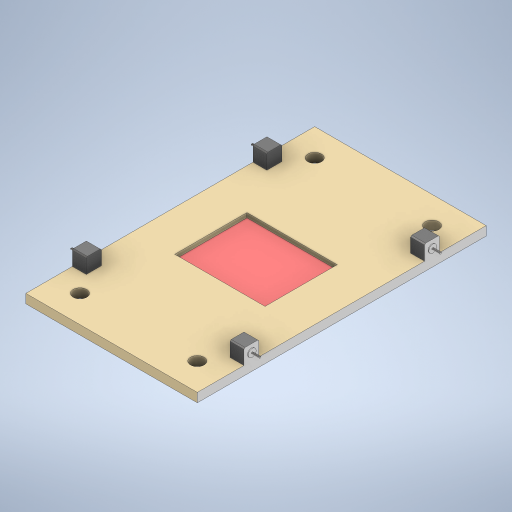
# Autodesk Inventor part: ChairBasePrototype
Saved by Autodesk Inventor 2023 (Build 270158000, 158)
## iProperties
Created: 2024-04-20
Part Number: ChairBasePrototype
Material: Generic
Document SubType Name: Modeling
Designer: andre
Density: 1 g/cm^3
Appearance: Default
Author: andre
Autodesk Inventor part; units mm, degrees
note: some values were not read from the file. Chosen so that the rebuilt part matches the saved one: pattern direction of "Rectangular Pattern1".
ref_plane "YZ Plane" through (0, 0, 0) normal (1, 0, 0) x (0, 1, 0)
ref_plane "XZ Plane" through (0, 0, 0) normal (0, 1, 0) x (-1, 0, 0)
ref_plane "XY Plane" through (0, 0, 0) normal (0, 0, 1) x (1, 0, 0)
sketch "Sketch1" plane through (0, 0, 0) normal (0, 1, 0) x (-1, 0, 0)
  line L0 (241.3, 406.4) -> (-241.3, 406.4)
  line L1 (-241.3, 406.4) -> (-241.3, -406.4)
  line L2 (-241.3, -406.4) -> (241.3, -406.4)
  line L3 (241.3, -406.4) -> (241.3, 406.4)
  line L4 (241.3, 406.4) -> (-241.3, -406.4) construction
  line L5 (-241.3, 406.4) -> (241.3, -406.4) construction
  point P0 (0, 0)
  dimension "d0" = 482.6
  dimension "d1" = 812.8
  constraints: 12 end point, 2 midpoint, 2 parallel, 1 horizontal, 1 perpendicular
  measures "d0" distance of L2.end L1.end
  measures "d1" distance of L1.end L0.end
extrude "Extrusion1" add sketch "Sketch1" along normal blind 25.4
sketch "Sketch2" plane through (0, 25.4, 0) normal (0, 1, 0) x (1, 0, 0)
  circle A0 centre (-165.1, 330.2) radius 19.05
  line L0 (-241.3, 406.4) -> (-241.3, -406.4) projected
  line L1 (241.3, 406.4) -> (-241.3, 406.4) projected
  circle A1 centre (165.1, 330.2) radius 19.05
  circle A2 centre (-165.1, -330.2) radius 19.05
  circle A3 centre (165.1, -330.2) radius 19.05
  line L2 (241.3, -406.4) -> (241.3, 406.4) projected
  line L3 (-241.3, -406.4) -> (241.3, -406.4) projected
  point P0 (0, 0)
  dimension "d4" = 38.1
  dimension "d5" = 76.2
  dimension "d6" = 76.2
  dimension "d9" = 38.1
  dimension "d10" = 38.1
  dimension "d11" = 38.1
  dimension "d12" = 76.2
  dimension "d13" = 76.2
  dimension "d14" = 76.2
  dimension "d15" = 76.2
  dimension "d16" = 76.2
  dimension "d17" = 76.2
  constraints: 4 centre point
  measures "d4" diameter of A0
  measures "d5" distance from line of L0 A0.centre
  measures "d6" distance from line of L1 A0.centre
  measures "d9" diameter of A1
  measures "d10" diameter of A2
  measures "d11" diameter of A3
  measures "d12" distance from line of L1 A1.centre
  measures "d13" distance from line of L2 A1.centre
  measures "d14" distance from line of L3 A3.centre
  measures "d15" distance from line of L2 A3.centre
  measures "d16" distance from line of L0 A2.centre
  measures "d17" distance from line of L3 A2.centre
extrude "Extrusion2" cut sketch "Sketch2" against normal blind 25.4 contours A0 | A1 | A2 | A3
sketch "Sketch3" plane through (0, 25.4, 0) normal (0, 1, 0) x (1, 0, 0)
  line L0 (-127, -101.6) -> (127, -101.6)
  line L1 (127, -101.6) -> (127, 101.6)
  line L2 (127, 101.6) -> (-127, 101.6)
  line L3 (-127, 101.6) -> (-127, -101.6)
  line L4 (-127, -101.6) -> (127, 101.6) construction
  line L5 (127, -101.6) -> (-127, 101.6) construction
  point P0 (0, 0)
  dimension "d18" = 254
  dimension "d19" = 203.2
  constraints: 12 end point, 2 midpoint, 2 parallel, 1 horizontal, 1 perpendicular
  measures "d18" distance of L2.end L1.end
  measures "d19" distance of L1.end L0.end
extrude "Extrusion3" cut sketch "Sketch3" against normal blind 12.7
sketch "Sketch4" plane through (0, 25.4, 0) normal (0, 1, 0) x (1, 0, 0)
  line L0 (241.3, -406.4) -> (241.3, 406.4) projected
  line L1 (241.3, -232.909) -> (202.3, -232.909)
  line L2 (202.3, -232.909) -> (202.3, -275.209)
  line L3 (202.3, -275.209) -> (241.3, -275.209)
  line L4 (241.3, -275.209) -> (241.3, -232.909)
  line L5 (127, -101.6) -> (-127, -101.6) projected
  line L6 (-241.3, -406.4) -> (241.3, -406.4) projected
  line L7 (-241.3, 406.4) -> (-241.3, -406.4) projected
  line L8 (-241.3, -232.909) -> (-202.3, -232.909)
  line L9 (-202.3, -232.909) -> (-202.3, -275.209)
  line L10 (-202.3, -275.209) -> (-241.3, -275.209)
  line L11 (-241.3, -275.209) -> (-241.3, -232.909)
  line L12 (-241.3, 275.209) -> (-202.3, 275.209)
  line L13 (-202.3, 275.209) -> (-202.3, 232.909)
  line L14 (-202.3, 232.909) -> (-241.3, 232.909)
  line L15 (-241.3, 232.909) -> (-241.3, 275.209)
  line L16 (241.3, 406.4) -> (-241.3, 406.4) projected
  line L17 (241.3, 275.209) -> (202.3, 275.209)
  line L18 (202.3, 275.209) -> (202.3, 232.909)
  line L19 (202.3, 232.909) -> (241.3, 232.909)
  line L20 (241.3, 232.909) -> (241.3, 275.209)
  point P0 (0, 0)
  point P1 (221.8, -232.909)
  point P2 (241.3, 232.909)
  point P3 (202.3, -254.059)
  point P4 (202.3, 254.059)
  dimension "d22" = 39
  dimension "d23" = 42.3
  dimension "d24" = 304.8
  dimension "d25" = 131.191
  dimension "d26" = 131.309
  dimension "d27" = 39
  dimension "d28" = 42.3
  dimension "d29" = 131.191
  dimension "d30" = 39
  dimension "d31" = 42.3
  dimension "d32" = 131.191
  dimension "d33" = 39
  dimension "d34" = 42.3
  dimension "d35" = 131.191
  dimension "d52" = 812.8
  dimension "d53" = 152.341
  dimension "d54" = 508.118
  constraints: 32 end point, 8 parallel, 4 horizontal, 4 perpendicular, 4 point on line, 3 midpoint
  measures "d22" distance of L3.end L2.end
  measures "d23" distance of L2.end L1.end
  measures "d24" distance between parallel lines of L5 L6
  measures "d25" distance between parallel lines of L6 L3
  measures "d26" distance from line of point (221.8, -232.909) L5
  measures "d27" distance of L9.end L10.end
  measures "d28" distance of L8.end L9.end
  measures "d29" distance between parallel lines of L6 L10
  measures "d30" distance of L13.end L14.end
  measures "d31" distance of L12.end L13.end
  measures "d32" distance between parallel lines of L16 L12
  measures "d33" distance of L19.end L18.end
  measures "d34" distance of L18.end L17.end
  measures "d35" distance between parallel lines of L16 L17
  measures "d52" distance between parallel lines of L6 L16
  measures "d53" distance from line of L6 point (202.3, -254.059)
  measures "d54" distance of point (202.3, -254.059) point (202.3, 254.059)
extrude "Extrusion4" add sketch "Sketch4" along normal blind 42.418 contours L3 L2 L1 L0 | L7 L8 L9 L10 | L19 L18 L17 L0 | L7 L12 L13 L14
sketch "Sketch5" plane through (241.3, 0, 406.4) normal (1, 0, 0) x (0, 0, -1)
  line L0 (0, 25.4) -> (131.191, 25.4) construction
  line L1 (173.491, 25.4) -> (639.309, 25.4) construction
  line L2 (131.191, 25.4) -> (173.491, 25.4) construction
  line L3 (131.191, 25.4) -> (131.191, 67.818) construction
  line L4 (173.491, 25.4) -> (131.191, 67.818) construction
  line L5 (173.491, 25.4) -> (173.491, 67.818) construction
  line L6 (173.491, 67.818) -> (131.191, 25.4) construction
  circle A0 centre (152.341, 46.609) radius 2.5273
  point P0 (406.4, 0)
  dimension "d38" = 5.0546
  constraints: 6 end point, 1 centre point, 1 horizontal, 1 midpoint
  measures "d38" diameter of A0
extrude "Extrusion5" add sketch "Sketch5" along normal blind 24.003
sketch "Sketch6" plane through (265.303, 46.609, 254.059) normal (1, 0, 0) x (0, 0, -1)
  line L0 (-3.2171, 1.2636) -> (4.0062, 1.2636)
  circle A0 centre (0, 0) radius 2.5273 projected
  point P0 (254.059, -46.609)
  point P1 (0, 2.5273)
  point P2 (0, -2.5273)
  point P3 (2.1887, 1.2636)
  point P4 (-2.1887, 1.2636)
  dimension "d42" = 5.0546
  dimension "d45" = 3.791
  constraints: 2 end point, 2 point on circle, 1 horizontal
  measures "d42" distance of A0.end A0.start
  measures "d45" distance from line of A0.end L0
extrude "Extrusion6" cut sketch "Sketch6" against normal blind 20 contours A0 L0 picked at (0.0978, 1.9929)
sketch "Sketch7" plane through (241.3, 0, 406.4) normal (1, 0, 0) x (0, 0, -1)
  circle A0 centre (152.341, 46.609) radius 11
  point P0 (406.4, 0)
  dimension "d46" = 22
  constraints: 1 centre point, 1 coincident
  measures "d46" diameter of A0
extrude "Extrusion7" add sketch "Sketch7" along normal blind 2
pattern_linear "Rectangular Pattern1" count 2 spacing 508.127 along (0, 0, -1) of "Extrusion7", "Extrusion6", "Extrusion5" first direction both ways yes
mirror "Mirror1" about plane through (0, 0, 0) normal (1, 0, 0) of "Extrusion7", "Extrusion6", "Extrusion5", "Rectangular Pattern1"
chamfer "Chamfer1" distance 3.175 angle 45 8 edges at (221.8, 67.818, 275.209) (221.8, 67.818, 232.909) (221.8, 67.818, -275.209) (221.8, 67.818, -232.909) (-221.8, 67.818, -275.209) (-221.8, 67.818, -232.909) (-221.8, 67.818, 232.909) (-221.8, 67.818, 275.209)
body "Solid1"
